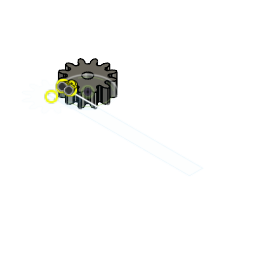
mechtasknipun (Autodesk Fusion 360 design; units mm, degrees)
part number: 2026-02-09-14-14-05-386
description: Spur Gear; Module: 2.1428; Num Teeth: 12; Pressure Angle: 20.0; Backlash: 0.00 mm
part number: 2026-02-09-14-34-28-587
Autodesk Fusion 360 part; units mm, degrees
(part 1 of 2)
sketch "Sketch1" plane through (0, 0, 0) normal (0, 0, 1) x (1, 0, 0)
  circle A0 centre (0, 0) radius 15
  dimension "d1" = 30
  constraint coincident A0.centre origin
  measures "d1" diameter of A0
sketch "Sketch1 (2)" plane through (0, 0, 0) normal (0, 0, 1) x (1, 0, 0) in component "Spur Gear (12 teeth)"
  circle A0 centre (0, 0) radius 10.2346
  circle A1 centre (0, 0) radius 3
extrude "Extrude1" add sketch "Sketch1 (2)" along normal blind 10 makes body 1 in component "Spur Gear (12 teeth)"
sketch "Sketch2" plane through (0, 0, 0) normal (0, 0, 1) x (1, 0, 0) in component "Spur Gear (12 teeth)"
  spline S0 degree 5 poles (11.9532, -1.7553) (11.9618, -1.7565) (11.979, -1.7588) (12.0048, -1.7613) (12.0394, -1.7631) (12.0828, -1.7633) (12.1263, -1.7619) (12.1699, -1.7595) (12.2135, -1.7567) (12.2572, -1.7535) (12.301, -1.7499) (12.3447, -1.7458) (12.3885, -1.741) (12.4324, -1.7355) (12.4763, -1.7292) (12.5202, -1.7222) (12.5641, -1.7147) (12.6081, -1.7066) (12.652, -1.698) (12.696, -1.6891) (12.74, -1.6797) (12.7839, -1.6698) (12.8279, -1.6595) (12.8719, -1.6487) (12.9159, -1.6374) (12.9598, -1.6257) (13.0038, -1.6135) (13.0477, -1.6009) (13.0916, -1.5879) (13.1355, -1.5745) (13.1794, -1.5607) (13.2233, -1.5466) (13.2671, -1.532) (13.311, -1.517) (13.3548, -1.5016) (13.3985, -1.4859) (13.4423, -1.4697) (13.486, -1.4532) (13.5297, -1.4364) (13.5733, -1.4192) (13.6169, -1.4016) (13.6605, -1.3836) (13.704, -1.3654) (13.7475, -1.3467) (13.791, -1.3277) (13.8344, -1.3084) (13.8778, -1.2887) (13.9211, -1.2687) (13.9643, -1.2483) (14.0076, -1.2277) (14.0507, -1.2066) (14.0939, -1.1853) (14.1369, -1.1636) (14.1799, -1.1416) (14.2229, -1.1193) (14.2658, -1.0967) (14.3086, -1.0738) (14.3514, -1.0505) (14.3941, -1.0269) (14.4367, -1.003) (14.4793, -0.9788) (14.5218, -0.9543) (14.5643, -0.9295) (14.6067, -0.9044) (14.649, -0.879) (14.6912, -0.8533) (14.7334, -0.8273) (14.7755, -0.801) (14.8175, -0.7744) (14.8595, -0.7475) (14.9014, -0.7203) (14.9348, -0.6983) (14.9598, -0.6817) (14.9765, -0.6706) (14.9849, -0.665) knots 0 0 0 0 0 0 0.01428571 0.02857143 0.04285714 0.05714286 0.07142857 0.08571429 0.1 0.11428571 0.12857143 0.14285714 0.15714286 0.17142857 0.18571429 0.2 0.21428571 0.22857143 0.24285714 0.25714286 0.27142857 0.28571429 0.3 0.31428571 0.32857143 0.34285714 0.35714286 0.37142857 0.38571429 0.4 0.41428571 0.42857143 0.44285714 0.45714286 0.47142857 0.48571429 0.5 0.51428571 0.52857143 0.54285714 0.55714286 0.57142857 0.58571429 0.6 0.61428571 0.62857143 0.64285714 0.65714286 0.67142857 0.68571429 0.7 0.71428571 0.72857143 0.74285714 0.75714286 0.77142857 0.78571429 0.8 0.81428571 0.82857143 0.84285714 0.85714286 0.87142857 0.88571429 0.9 0.91428571 0.92857143 0.94285714 0.95714286 0.97142857 0.98571429 1 1 1 1 1 1
  spline S1 degree 5 poles (11.9532, 1.7553) (11.9618, 1.7565) (11.979, 1.7588) (12.0048, 1.7613) (12.0394, 1.7631) (12.0828, 1.7633) (12.1263, 1.7619) (12.1699, 1.7595) (12.2135, 1.7567) (12.2572, 1.7535) (12.301, 1.7499) (12.3447, 1.7458) (12.3885, 1.741) (12.4324, 1.7355) (12.4763, 1.7292) (12.5202, 1.7222) (12.5641, 1.7147) (12.6081, 1.7066) (12.652, 1.698) (12.696, 1.6891) (12.74, 1.6797) (12.7839, 1.6698) (12.8279, 1.6595) (12.8719, 1.6487) (12.9159, 1.6374) (12.9598, 1.6257) (13.0038, 1.6135) (13.0477, 1.6009) (13.0916, 1.5879) (13.1355, 1.5745) (13.1794, 1.5607) (13.2233, 1.5466) (13.2671, 1.532) (13.311, 1.517) (13.3548, 1.5016) (13.3985, 1.4859) (13.4423, 1.4697) (13.486, 1.4532) (13.5297, 1.4364) (13.5733, 1.4192) (13.6169, 1.4016) (13.6605, 1.3836) (13.704, 1.3654) (13.7475, 1.3467) (13.791, 1.3277) (13.8344, 1.3084) (13.8778, 1.2887) (13.9211, 1.2687) (13.9643, 1.2483) (14.0076, 1.2277) (14.0507, 1.2066) (14.0939, 1.1853) (14.1369, 1.1636) (14.1799, 1.1416) (14.2229, 1.1193) (14.2658, 1.0967) (14.3086, 1.0738) (14.3514, 1.0505) (14.3941, 1.0269) (14.4367, 1.003) (14.4793, 0.9788) (14.5218, 0.9543) (14.5643, 0.9295) (14.6067, 0.9044) (14.649, 0.879) (14.6912, 0.8533) (14.7334, 0.8273) (14.7755, 0.801) (14.8175, 0.7744) (14.8595, 0.7475) (14.9014, 0.7203) (14.9348, 0.6983) (14.9598, 0.6817) (14.9765, 0.6706) (14.9849, 0.665) knots 0 0 0 0 0 0 0.01428571 0.02857143 0.04285714 0.05714286 0.07142857 0.08571429 0.1 0.11428571 0.12857143 0.14285714 0.15714286 0.17142857 0.18571429 0.2 0.21428571 0.22857143 0.24285714 0.25714286 0.27142857 0.28571429 0.3 0.31428571 0.32857143 0.34285714 0.35714286 0.37142857 0.38571429 0.4 0.41428571 0.42857143 0.44285714 0.45714286 0.47142857 0.48571429 0.5 0.51428571 0.52857143 0.54285714 0.55714286 0.57142857 0.58571429 0.6 0.61428571 0.62857143 0.64285714 0.65714286 0.67142857 0.68571429 0.7 0.71428571 0.72857143 0.74285714 0.75714286 0.77142857 0.78571429 0.8 0.81428571 0.82857143 0.84285714 0.85714286 0.87142857 0.88571429 0.9 0.91428571 0.92857143 0.94285714 0.95714286 0.97142857 0.98571429 1 1 1 1 1 1
  arc A0 (14.9849, -0.665) -> (14.9849, 0.665) centre (0, 0) ccw
  line L0 (10.1162, -1.487) -> (11.9532, -1.7553)
  line L1 (10.1162, 1.487) -> (11.9532, 1.7553)
  line L2 (10.1162, -1.487) -> (10.1162, 1.487)
  point P0 (12.1632, -1.7598)
  point P1 (12.3763, -1.7422)
  point P2 (12.5912, -1.7096)
  point P3 (12.8075, -1.6642)
  point P4 (13.0248, -1.6074)
  point P5 (13.2428, -1.54)
  point P6 (13.4613, -1.4625)
  point P7 (13.68, -1.3754)
  point P8 (13.8987, -1.279)
  point P9 (14.1171, -1.1735)
  point P10 (14.3352, -1.0592)
  point P11 (14.5526, -0.9363)
  point P12 (14.7692, -0.8048)
  point P13 (12.1632, 1.7598)
  point P14 (12.3763, 1.7422)
  point P15 (12.5912, 1.7096)
  point P16 (12.8075, 1.6642)
  point P17 (13.0248, 1.6074)
  point P18 (13.2428, 1.54)
  point P19 (13.4613, 1.4625)
  point P20 (13.68, 1.3754)
  point P21 (13.8987, 1.279)
  point P22 (14.1171, 1.1735)
  point P23 (14.3352, 1.0592)
  point P24 (14.5526, 0.9363)
  point P25 (14.7692, 0.8048)
extrude "Extrude2" add sketch "Sketch2" along normal blind 10 bodies 1 in component "Spur Gear (12 teeth)"
fillet "Fillet1" radius 0.9 2 edges at (10.1258, -1.4884, 5) (10.1258, 1.4884, 5) on bodies 1 in component "Spur Gear (12 teeth)"
pattern_circular "C-Pattern1" count 12 over 360 about axis through (0, 0, 0) along (0, 0, 1) of "Extrude2", "Fillet1" in component "Spur Gear (12 teeth)"
sketch "Sketch3" plane through (0, 0, 0) normal (0, 0, 1) x (1, 0, 0) in component "Spur Gear (12 teeth)"
  circle A0 centre (0, 0) radius 12.8568 construction
copy_body "CopyPasteBodies1" bodies 1 makes body 2
move_body "Move1" bodies 2 to x (1, 0, 0) y (0, 1, 0) z (0, 0, 1) at (0, 0, 0)
sketch "Sketch2 (2)" plane through (0, 0, 10) normal (0, 0, 1) x (-1, 0, 0)
  arc A0 (-9.7871, 28.7076) -> (-9.9726, 28.0156) centre (0, 25.7143) ccw
  arc A1 (-10.9796, 27.3274) -> (-9.9726, 28.0156) centre (-10.8495, 28.2179) ccw
  line L0 (-10.9796, 27.3274) -> (-11.9532, 27.4696)
  spline S0 degree 5 poles (-11.9532, 27.4696) (-11.9618, 27.4708) (-11.979, 27.4731) (-12.0048, 27.4756) (-12.0394, 27.4774) (-12.0828, 27.4775) (-12.1263, 27.4762) (-12.1699, 27.4738) (-12.2135, 27.471) (-12.2572, 27.4677) (-12.301, 27.4642) (-12.3447, 27.4601) (-12.3885, 27.4553) (-12.4324, 27.4498) (-12.4763, 27.4435) (-12.5202, 27.4365) (-12.5641, 27.4289) (-12.6081, 27.4208) (-12.652, 27.4123) (-12.696, 27.4033) (-12.74, 27.394) (-12.7839, 27.3841) (-12.8279, 27.3738) (-12.8719, 27.363) (-12.9159, 27.3517) (-12.9598, 27.34) (-13.0038, 27.3278) (-13.0477, 27.3152) (-13.0916, 27.3022) (-13.1355, 27.2888) (-13.1794, 27.275) (-13.2233, 27.2608) (-13.2671, 27.2463) (-13.311, 27.2313) (-13.3548, 27.2159) (-13.3985, 27.2002) (-13.4423, 27.184) (-13.486, 27.1675) (-13.5297, 27.1507) (-13.5733, 27.1334) (-13.6169, 27.1159) (-13.6605, 27.0979) (-13.704, 27.0796) (-13.7475, 27.061) (-13.791, 27.042) (-13.8344, 27.0227) (-13.8778, 27.003) (-13.9211, 26.983) (-13.9643, 26.9626) (-14.0076, 26.9419) (-14.0507, 26.9209) (-14.0939, 26.8996) (-14.1369, 26.8779) (-14.1799, 26.8559) (-14.2229, 26.8336) (-14.2658, 26.811) (-14.3086, 26.788) (-14.3514, 26.7648) (-14.3941, 26.7412) (-14.4367, 26.7173) (-14.4793, 26.6931) (-14.5218, 26.6686) (-14.5643, 26.6438) (-14.6067, 26.6187) (-14.649, 26.5933) (-14.6912, 26.5676) (-14.7334, 26.5416) (-14.7755, 26.5153) (-14.8175, 26.4887) (-14.8595, 26.4618) (-14.9014, 26.4346) (-14.9348, 26.4126) (-14.9598, 26.396) (-14.9765, 26.3849) (-14.9849, 26.3793) knots 0 0 0 0 0 0 0.01428571 0.02857143 0.04285714 0.05714286 0.07142857 0.08571429 0.1 0.11428571 0.12857143 0.14285714 0.15714286 0.17142857 0.18571429 0.2 0.21428571 0.22857143 0.24285714 0.25714286 0.27142857 0.28571429 0.3 0.31428571 0.32857143 0.34285714 0.35714286 0.37142857 0.38571429 0.4 0.41428571 0.42857143 0.44285714 0.45714286 0.47142857 0.48571429 0.5 0.51428571 0.52857143 0.54285714 0.55714286 0.57142857 0.58571429 0.6 0.61428571 0.62857143 0.64285714 0.65714286 0.67142857 0.68571429 0.7 0.71428571 0.72857143 0.74285714 0.75714286 0.77142857 0.78571429 0.8 0.81428571 0.82857143 0.84285714 0.85714286 0.87142857 0.88571429 0.9 0.91428571 0.92857143 0.94285714 0.95714286 0.97142857 0.98571429 1 1 1 1 1 1
  arc A2 (-14.9849, 26.3793) -> (-14.9849, 25.0493) centre (0, 25.7143) ccw
  spline S1 degree 5 poles (-14.9849, 25.0493) (-14.9765, 25.0437) (-14.9598, 25.0326) (-14.9348, 25.0159) (-14.9014, 24.994) (-14.8595, 24.9668) (-14.8175, 24.9399) (-14.7755, 24.9133) (-14.7334, 24.887) (-14.6912, 24.861) (-14.649, 24.8353) (-14.6067, 24.8099) (-14.5643, 24.7847) (-14.5218, 24.7599) (-14.4793, 24.7354) (-14.4367, 24.7112) (-14.3941, 24.6874) (-14.3514, 24.6638) (-14.3086, 24.6405) (-14.2658, 24.6176) (-14.2229, 24.5949) (-14.1799, 24.5726) (-14.1369, 24.5506) (-14.0939, 24.529) (-14.0507, 24.5076) (-14.0076, 24.4866) (-13.9643, 24.4659) (-13.9211, 24.4456) (-13.8778, 24.4256) (-13.8344, 24.4059) (-13.791, 24.3866) (-13.7475, 24.3676) (-13.704, 24.3489) (-13.6605, 24.3306) (-13.6169, 24.3127) (-13.5733, 24.2951) (-13.5297, 24.2779) (-13.486, 24.261) (-13.4423, 24.2445) (-13.3985, 24.2284) (-13.3548, 24.2127) (-13.311, 24.1973) (-13.2671, 24.1823) (-13.2233, 24.1677) (-13.1794, 24.1535) (-13.1355, 24.1398) (-13.0916, 24.1264) (-13.0477, 24.1134) (-13.0038, 24.1008) (-12.9598, 24.0886) (-12.9159, 24.0768) (-12.8719, 24.0656) (-12.8279, 24.0548) (-12.7839, 24.0445) (-12.74, 24.0346) (-12.696, 24.0252) (-12.652, 24.0163) (-12.6081, 24.0077) (-12.5641, 23.9996) (-12.5202, 23.992) (-12.4763, 23.9851) (-12.4324, 23.9788) (-12.3885, 23.9733) (-12.3447, 23.9685) (-12.301, 23.9644) (-12.2572, 23.9608) (-12.2135, 23.9576) (-12.1699, 23.9548) (-12.1263, 23.9524) (-12.0828, 23.951) (-12.0394, 23.9512) (-12.0048, 23.953) (-11.979, 23.9555) (-11.9618, 23.9577) (-11.9532, 23.959) knots -1 -1 -1 -1 -1 -1 -0.98571429 -0.97142857 -0.95714286 -0.94285714 -0.92857143 -0.91428571 -0.9 -0.88571429 -0.87142857 -0.85714286 -0.84285714 -0.82857143 -0.81428571 -0.8 -0.78571429 -0.77142857 -0.75714286 -0.74285714 -0.72857143 -0.71428571 -0.7 -0.68571429 -0.67142857 -0.65714286 -0.64285714 -0.62857143 -0.61428571 -0.6 -0.58571429 -0.57142857 -0.55714286 -0.54285714 -0.52857143 -0.51428571 -0.5 -0.48571429 -0.47142857 -0.45714286 -0.44285714 -0.42857143 -0.41428571 -0.4 -0.38571429 -0.37142857 -0.35714286 -0.34285714 -0.32857143 -0.31428571 -0.3 -0.28571429 -0.27142857 -0.25714286 -0.24285714 -0.22857143 -0.21428571 -0.2 -0.18571429 -0.17142857 -0.15714286 -0.14285714 -0.12857143 -0.11428571 -0.1 -0.08571429 -0.07142857 -0.05714286 -0.04285714 -0.02857143 -0.01428571 0 0 0 0 0 0
  line L1 (-11.9532, 23.959) -> (-10.9796, 24.1012)
  arc A3 (-9.9726, 23.413) -> (-10.9796, 24.1012) centre (-10.8495, 23.2107) ccw
  arc A4 (-9.9726, 23.413) -> (-9.7871, 22.721) centre (0, 25.7143) ccw
  arc A5 (-10.3151, 21.6215) -> (-9.7871, 22.721) centre (-10.6478, 22.4577) ccw
  line L2 (-10.3151, 21.6215) -> (-11.2295, 21.2578)
  spline S2 degree 5 poles (-11.2295, 21.2578) (-11.2375, 21.2546) (-11.2535, 21.2479) (-11.2771, 21.2372) (-11.308, 21.2215) (-11.3456, 21.1999) (-11.3826, 21.177) (-11.4192, 21.1532) (-11.4556, 21.1289) (-11.4918, 21.1042) (-11.5279, 21.0792) (-11.5637, 21.0538) (-11.5993, 21.0278) (-11.6345, 21.0011) (-11.6694, 20.9737) (-11.7039, 20.9457) (-11.7382, 20.9172) (-11.7722, 20.8882) (-11.806, 20.8588) (-11.8396, 20.8291) (-11.873, 20.7989) (-11.9061, 20.7684) (-11.9391, 20.7375) (-11.9717, 20.7062) (-12.0042, 20.6744) (-12.0364, 20.6423) (-12.0684, 20.6098) (-12.1001, 20.5769) (-12.1316, 20.5437) (-12.163, 20.5101) (-12.1941, 20.4762) (-12.225, 20.442) (-12.2557, 20.4074) (-12.2861, 20.3726) (-12.3164, 20.3373) (-12.3464, 20.3018) (-12.3762, 20.266) (-12.4058, 20.2298) (-12.4352, 20.1934) (-12.4644, 20.1567) (-12.4934, 20.1196) (-12.5222, 20.0823) (-12.5507, 20.0447) (-12.5791, 20.0068) (-12.6072, 19.9686) (-12.6351, 19.9302) (-12.6628, 19.8915) (-12.6904, 19.8525) (-12.7176, 19.8132) (-12.7447, 19.7737) (-12.7716, 19.7339) (-12.7983, 19.6939) (-12.8247, 19.6536) (-12.851, 19.613) (-12.877, 19.5722) (-12.9029, 19.5312) (-12.9285, 19.4899) (-12.9539, 19.4484) (-12.9791, 19.4066) (-13.0041, 19.3646) (-13.0289, 19.3223) (-13.0535, 19.2799) (-13.0778, 19.2371) (-13.102, 19.1942) (-13.1259, 19.151) (-13.1496, 19.1077) (-13.1732, 19.064) (-13.1965, 19.0202) (-13.2196, 18.9762) (-13.2424, 18.9319) (-13.2651, 18.8874) (-13.2831, 18.8517) (-13.2965, 18.8248) (-13.3053, 18.8068) (-13.3098, 18.7978) knots 0 0 0 0 0 0 0.01428571 0.02857143 0.04285714 0.05714286 0.07142857 0.08571429 0.1 0.11428571 0.12857143 0.14285714 0.15714286 0.17142857 0.18571429 0.2 0.21428571 0.22857143 0.24285714 0.25714286 0.27142857 0.28571429 0.3 0.31428571 0.32857143 0.34285714 0.35714286 0.37142857 0.38571429 0.4 0.41428571 0.42857143 0.44285714 0.45714286 0.47142857 0.48571429 0.5 0.51428571 0.52857143 0.54285714 0.55714286 0.57142857 0.58571429 0.6 0.61428571 0.62857143 0.64285714 0.65714286 0.67142857 0.68571429 0.7 0.71428571 0.72857143 0.74285714 0.75714286 0.77142857 0.78571429 0.8 0.81428571 0.82857143 0.84285714 0.85714286 0.87142857 0.88571429 0.9 0.91428571 0.92857143 0.94285714 0.95714286 0.97142857 0.98571429 1 1 1 1 1 1
  arc A6 (-13.3098, 18.7978) -> (-12.6448, 17.6459) centre (0, 25.7143) ccw
  spline S3 degree 5 poles (-12.6448, 17.6459) (-12.6347, 17.6453) (-12.6147, 17.644) (-12.5847, 17.6421) (-12.5448, 17.6398) (-12.4949, 17.6372) (-12.4452, 17.6349) (-12.3955, 17.6328) (-12.3459, 17.6311) (-12.2963, 17.6297) (-12.2469, 17.6285) (-12.1975, 17.6277) (-12.1483, 17.6271) (-12.0991, 17.6269) (-12.05, 17.6269) (-12.0011, 17.6273) (-11.9522, 17.6279) (-11.9034, 17.6288) (-11.8547, 17.6301) (-11.8062, 17.6316) (-11.7577, 17.6335) (-11.7093, 17.6356) (-11.6611, 17.6381) (-11.613, 17.6409) (-11.565, 17.6439) (-11.5171, 17.6473) (-11.4693, 17.651) (-11.4217, 17.655) (-11.3741, 17.6594) (-11.3267, 17.664) (-11.2795, 17.669) (-11.2324, 17.6742) (-11.1854, 17.6798) (-11.1385, 17.6858) (-11.0918, 17.692) (-11.0453, 17.6986) (-10.9989, 17.7055) (-10.9526, 17.7127) (-10.9065, 17.7203) (-10.8605, 17.7282) (-10.8148, 17.7365) (-10.7691, 17.745) (-10.7237, 17.754) (-10.6784, 17.7633) (-10.6334, 17.7729) (-10.5884, 17.7829) (-10.5437, 17.7933) (-10.4992, 17.804) (-10.4548, 17.815) (-10.4107, 17.8265) (-10.3667, 17.8383) (-10.323, 17.8505) (-10.2795, 17.8631) (-10.2363, 17.8762) (-10.1933, 17.8897) (-10.1505, 17.9035) (-10.108, 17.9177) (-10.0656, 17.9323) (-10.0235, 17.9473) (-9.9817, 17.9627) (-9.9402, 17.9786) (-9.899, 17.9951) (-9.8583, 18.0123) (-9.818, 18.03) (-9.778, 18.0484) (-9.7383, 18.0671) (-9.6989, 18.0862) (-9.6596, 18.1056) (-9.6207, 18.1253) (-9.5823, 18.1459) (-9.5448, 18.1677) (-9.5158, 18.1865) (-9.4947, 18.2016) (-9.481, 18.2122) (-9.4742, 18.2175) knots -1 -1 -1 -1 -1 -1 -0.98571429 -0.97142857 -0.95714286 -0.94285714 -0.92857143 -0.91428571 -0.9 -0.88571429 -0.87142857 -0.85714286 -0.84285714 -0.82857143 -0.81428571 -0.8 -0.78571429 -0.77142857 -0.75714286 -0.74285714 -0.72857143 -0.71428571 -0.7 -0.68571429 -0.67142857 -0.65714286 -0.64285714 -0.62857143 -0.61428571 -0.6 -0.58571429 -0.57142857 -0.55714286 -0.54285714 -0.52857143 -0.51428571 -0.5 -0.48571429 -0.47142857 -0.45714286 -0.44285714 -0.42857143 -0.41428571 -0.4 -0.38571429 -0.37142857 -0.35714286 -0.34285714 -0.32857143 -0.31428571 -0.3 -0.28571429 -0.27142857 -0.25714286 -0.24285714 -0.22857143 -0.21428571 -0.2 -0.18571429 -0.17142857 -0.15714286 -0.14285714 -0.12857143 -0.11428571 -0.1 -0.08571429 -0.07142857 -0.05714286 -0.04285714 -0.02857143 -0.01428571 0 0 0 0 0 0
  line L3 (-9.4742, 18.2175) -> (-8.7021, 18.8275)
  arc A7 (-7.4859, 18.735) -> (-8.7021, 18.8275) centre (-8.1441, 18.1213) ccw
  arc A8 (-7.4859, 18.735) -> (-6.9792, 18.2284) centre (0, 25.7143) ccw
  arc A9 (-6.8868, 17.0122) -> (-6.9792, 18.2284) centre (-7.593, 17.5701) ccw
  line L4 (-6.8868, 17.0122) -> (-7.4967, 16.2401)
  spline S4 degree 5 poles (-7.4967, 16.2401) (-7.5021, 16.2333) (-7.5126, 16.2196) (-7.5277, 16.1985) (-7.5466, 16.1694) (-7.5684, 16.1319) (-7.589, 16.0936) (-7.6087, 16.0546) (-7.6281, 16.0154) (-7.6472, 15.976) (-7.6659, 15.9363) (-7.6842, 15.8963) (-7.702, 15.856) (-7.7192, 15.8153) (-7.7357, 15.7741) (-7.7516, 15.7326) (-7.767, 15.6908) (-7.782, 15.6486) (-7.7966, 15.6063) (-7.8108, 15.5638) (-7.8246, 15.521) (-7.8381, 15.478) (-7.8511, 15.4347) (-7.8638, 15.3913) (-7.876, 15.3475) (-7.8878, 15.3036) (-7.8992, 15.2595) (-7.9103, 15.2151) (-7.921, 15.1706) (-7.9314, 15.1258) (-7.9414, 15.0809) (-7.951, 15.0358) (-7.9603, 14.9906) (-7.9692, 14.9451) (-7.9778, 14.8995) (-7.9861, 14.8537) (-7.994, 14.8078) (-8.0016, 14.7617) (-8.0088, 14.7154) (-8.0157, 14.669) (-8.0223, 14.6225) (-8.0285, 14.5758) (-8.0345, 14.5289) (-8.0401, 14.4819) (-8.0453, 14.4348) (-8.0503, 14.3875) (-8.0549, 14.3401) (-8.0593, 14.2926) (-8.0633, 14.245) (-8.067, 14.1972) (-8.0704, 14.1493) (-8.0734, 14.1013) (-8.0762, 14.0532) (-8.0787, 14.0049) (-8.0808, 13.9566) (-8.0827, 13.9081) (-8.0842, 13.8596) (-8.0854, 13.8109) (-8.0864, 13.7621) (-8.087, 13.7132) (-8.0874, 13.6643) (-8.0874, 13.6152) (-8.0871, 13.566) (-8.0866, 13.5167) (-8.0857, 13.4674) (-8.0846, 13.418) (-8.0832, 13.3684) (-8.0814, 13.3188) (-8.0794, 13.2691) (-8.0771, 13.2194) (-8.0745, 13.1695) (-8.0722, 13.1296) (-8.0703, 13.0996) (-8.069, 13.0795) (-8.0683, 13.0695) knots 0 0 0 0 0 0 0.01428571 0.02857143 0.04285714 0.05714286 0.07142857 0.08571429 0.1 0.11428571 0.12857143 0.14285714 0.15714286 0.17142857 0.18571429 0.2 0.21428571 0.22857143 0.24285714 0.25714286 0.27142857 0.28571429 0.3 0.31428571 0.32857143 0.34285714 0.35714286 0.37142857 0.38571429 0.4 0.41428571 0.42857143 0.44285714 0.45714286 0.47142857 0.48571429 0.5 0.51428571 0.52857143 0.54285714 0.55714286 0.57142857 0.58571429 0.6 0.61428571 0.62857143 0.64285714 0.65714286 0.67142857 0.68571429 0.7 0.71428571 0.72857143 0.74285714 0.75714286 0.77142857 0.78571429 0.8 0.81428571 0.82857143 0.84285714 0.85714286 0.87142857 0.88571429 0.9 0.91428571 0.92857143 0.94285714 0.95714286 0.97142857 0.98571429 1 1 1 1 1 1
  arc A10 (-8.0683, 13.0695) -> (-6.9165, 12.4045) centre (0, 25.7143) ccw
  spline S5 degree 5 poles (-6.9165, 12.4045) (-6.9075, 12.4089) (-6.8895, 12.4178) (-6.8626, 12.4312) (-6.8269, 12.4492) (-6.7824, 12.4718) (-6.7381, 12.4947) (-6.6941, 12.5178) (-6.6502, 12.5411) (-6.6066, 12.5646) (-6.5632, 12.5884) (-6.5201, 12.6123) (-6.4771, 12.6365) (-6.4344, 12.6608) (-6.392, 12.6854) (-6.3497, 12.7102) (-6.3077, 12.7352) (-6.2659, 12.7604) (-6.2244, 12.7858) (-6.1831, 12.8114) (-6.1421, 12.8372) (-6.1013, 12.8633) (-6.0607, 12.8895) (-6.0204, 12.916) (-5.9804, 12.9427) (-5.9406, 12.9695) (-5.9011, 12.9966) (-5.8618, 13.0239) (-5.8228, 13.0514) (-5.7841, 13.0792) (-5.7457, 13.1071) (-5.7075, 13.1352) (-5.6696, 13.1636) (-5.632, 13.1921) (-5.5947, 13.2209) (-5.5576, 13.2499) (-5.5209, 13.279) (-5.4845, 13.3084) (-5.4483, 13.338) (-5.4125, 13.3679) (-5.3769, 13.3979) (-5.3417, 13.4281) (-5.3068, 13.4586) (-5.2723, 13.4893) (-5.2381, 13.5202) (-5.2042, 13.5513) (-5.1706, 13.5826) (-5.1374, 13.6142) (-5.1045, 13.6459) (-5.072, 13.6779) (-5.0399, 13.7101) (-5.0081, 13.7425) (-4.9768, 13.7752) (-4.9459, 13.8081) (-4.9153, 13.8413) (-4.8852, 13.8747) (-4.8555, 13.9083) (-4.8261, 13.9421) (-4.7971, 13.9761) (-4.7686, 14.0104) (-4.7406, 14.0449) (-4.7132, 14.0798) (-4.6865, 14.115) (-4.6605, 14.1506) (-4.635, 14.1864) (-4.6101, 14.2225) (-4.5854, 14.2587) (-4.5611, 14.2951) (-4.5373, 14.3317) (-4.5143, 14.3687) (-4.4928, 14.4063) (-4.4771, 14.4372) (-4.4664, 14.4608) (-4.4597, 14.4768) (-4.4565, 14.4848) knots -1 -1 -1 -1 -1 -1 -0.98571429 -0.97142857 -0.95714286 -0.94285714 -0.92857143 -0.91428571 -0.9 -0.88571429 -0.87142857 -0.85714286 -0.84285714 -0.82857143 -0.81428571 -0.8 -0.78571429 -0.77142857 -0.75714286 -0.74285714 -0.72857143 -0.71428571 -0.7 -0.68571429 -0.67142857 -0.65714286 -0.64285714 -0.62857143 -0.61428571 -0.6 -0.58571429 -0.57142857 -0.55714286 -0.54285714 -0.52857143 -0.51428571 -0.5 -0.48571429 -0.47142857 -0.45714286 -0.44285714 -0.42857143 -0.41428571 -0.4 -0.38571429 -0.37142857 -0.35714286 -0.34285714 -0.32857143 -0.31428571 -0.3 -0.28571429 -0.27142857 -0.25714286 -0.24285714 -0.22857143 -0.21428571 -0.2 -0.18571429 -0.17142857 -0.15714286 -0.14285714 -0.12857143 -0.11428571 -0.1 -0.08571429 -0.07142857 -0.05714286 -0.04285714 -0.02857143 -0.01428571 0 0 0 0 0 0
  line L5 (-4.4565, 14.4848) -> (-4.0928, 15.3991)
  arc A11 (-2.9933, 15.9272) -> (-4.0928, 15.3991) centre (-3.2566, 15.0665) ccw
  arc A12 (-2.9933, 15.9272) -> (-2.3013, 15.7417) centre (0, 25.7143) ccw
  arc A13 (-1.6131, 14.7347) -> (-2.3013, 15.7417) centre (-2.5036, 14.8648) ccw
  line L6 (-1.6131, 14.7347) -> (-1.7553, 13.761)
  spline S6 degree 5 poles (-1.7553, 13.761) (-1.7565, 13.7525) (-1.7588, 13.7353) (-1.7613, 13.7095) (-1.7631, 13.6749) (-1.7633, 13.6315) (-1.7619, 13.588) (-1.7595, 13.5444) (-1.7567, 13.5008) (-1.7535, 13.4571) (-1.7499, 13.4133) (-1.7458, 13.3696) (-1.741, 13.3257) (-1.7355, 13.2819) (-1.7292, 13.238) (-1.7222, 13.1941) (-1.7147, 13.1502) (-1.7066, 13.1062) (-1.698, 13.0622) (-1.6891, 13.0183) (-1.6797, 12.9743) (-1.6698, 12.9303) (-1.6595, 12.8864) (-1.6487, 12.8424) (-1.6374, 12.7984) (-1.6257, 12.7545) (-1.6135, 12.7105) (-1.6009, 12.6666) (-1.5879, 12.6227) (-1.5745, 12.5787) (-1.5607, 12.5349) (-1.5466, 12.491) (-1.532, 12.4471) (-1.517, 12.4033) (-1.5016, 12.3595) (-1.4859, 12.3157) (-1.4697, 12.272) (-1.4532, 12.2283) (-1.4364, 12.1846) (-1.4192, 12.141) (-1.4016, 12.0973) (-1.3836, 12.0538) (-1.3654, 12.0102) (-1.3467, 11.9667) (-1.3277, 11.9233) (-1.3084, 11.8799) (-1.2887, 11.8365) (-1.2687, 11.7932) (-1.2483, 11.7499) (-1.2277, 11.7067) (-1.2066, 11.6636) (-1.1853, 11.6204) (-1.1636, 11.5774) (-1.1416, 11.5344) (-1.1193, 11.4914) (-1.0967, 11.4485) (-1.0738, 11.4057) (-1.0505, 11.3629) (-1.0269, 11.3202) (-1.003, 11.2776) (-0.9788, 11.235) (-0.9543, 11.1924) (-0.9295, 11.15) (-0.9044, 11.1076) (-0.879, 11.0653) (-0.8533, 11.023) (-0.8273, 10.9809) (-0.801, 10.9388) (-0.7744, 10.8968) (-0.7475, 10.8548) (-0.7203, 10.8129) (-0.6983, 10.7795) (-0.6817, 10.7545) (-0.6706, 10.7378) (-0.665, 10.7294) knots 0 0 0 0 0 0 0.01428571 0.02857143 0.04285714 0.05714286 0.07142857 0.08571429 0.1 0.11428571 0.12857143 0.14285714 0.15714286 0.17142857 0.18571429 0.2 0.21428571 0.22857143 0.24285714 0.25714286 0.27142857 0.28571429 0.3 0.31428571 0.32857143 0.34285714 0.35714286 0.37142857 0.38571429 0.4 0.41428571 0.42857143 0.44285714 0.45714286 0.47142857 0.48571429 0.5 0.51428571 0.52857143 0.54285714 0.55714286 0.57142857 0.58571429 0.6 0.61428571 0.62857143 0.64285714 0.65714286 0.67142857 0.68571429 0.7 0.71428571 0.72857143 0.74285714 0.75714286 0.77142857 0.78571429 0.8 0.81428571 0.82857143 0.84285714 0.85714286 0.87142857 0.88571429 0.9 0.91428571 0.92857143 0.94285714 0.95714286 0.97142857 0.98571429 1 1 1 1 1 1
  arc A14 (-0.665, 10.7294) -> (0.665, 10.7294) centre (0, 25.7143) ccw
  spline S7 degree 5 poles (0.665, 10.7294) (0.6706, 10.7378) (0.6817, 10.7545) (0.6983, 10.7795) (0.7203, 10.8129) (0.7475, 10.8548) (0.7744, 10.8968) (0.801, 10.9388) (0.8273, 10.9809) (0.8533, 11.023) (0.879, 11.0653) (0.9044, 11.1076) (0.9295, 11.15) (0.9543, 11.1924) (0.9788, 11.235) (1.003, 11.2776) (1.0269, 11.3202) (1.0505, 11.3629) (1.0738, 11.4057) (1.0967, 11.4485) (1.1193, 11.4914) (1.1416, 11.5344) (1.1636, 11.5774) (1.1853, 11.6204) (1.2066, 11.6636) (1.2277, 11.7067) (1.2483, 11.7499) (1.2687, 11.7932) (1.2887, 11.8365) (1.3084, 11.8799) (1.3277, 11.9233) (1.3467, 11.9667) (1.3654, 12.0102) (1.3836, 12.0538) (1.4016, 12.0973) (1.4192, 12.141) (1.4364, 12.1846) (1.4532, 12.2283) (1.4697, 12.272) (1.4859, 12.3157) (1.5016, 12.3595) (1.517, 12.4033) (1.532, 12.4471) (1.5466, 12.491) (1.5607, 12.5349) (1.5745, 12.5787) (1.5879, 12.6227) (1.6009, 12.6666) (1.6135, 12.7105) (1.6257, 12.7545) (1.6374, 12.7984) (1.6487, 12.8424) (1.6595, 12.8864) (1.6698, 12.9303) (1.6797, 12.9743) (1.6891, 13.0183) (1.698, 13.0622) (1.7066, 13.1062) (1.7147, 13.1502) (1.7222, 13.1941) (1.7292, 13.238) (1.7355, 13.2819) (1.741, 13.3257) (1.7458, 13.3696) (1.7499, 13.4133) (1.7535, 13.4571) (1.7567, 13.5008) (1.7595, 13.5444) (1.7619, 13.588) (1.7633, 13.6315) (1.7631, 13.6749) (1.7613, 13.7095) (1.7588, 13.7353) (1.7565, 13.7525) (1.7553, 13.761) knots -1 -1 -1 -1 -1 -1 -0.98571429 -0.97142857 -0.95714286 -0.94285714 -0.92857143 -0.91428571 -0.9 -0.88571429 -0.87142857 -0.85714286 -0.84285714 -0.82857143 -0.81428571 -0.8 -0.78571429 -0.77142857 -0.75714286 -0.74285714 -0.72857143 -0.71428571 -0.7 -0.68571429 -0.67142857 -0.65714286 -0.64285714 -0.62857143 -0.61428571 -0.6 -0.58571429 -0.57142857 -0.55714286 -0.54285714 -0.52857143 -0.51428571 -0.5 -0.48571429 -0.47142857 -0.45714286 -0.44285714 -0.42857143 -0.41428571 -0.4 -0.38571429 -0.37142857 -0.35714286 -0.34285714 -0.32857143 -0.31428571 -0.3 -0.28571429 -0.27142857 -0.25714286 -0.24285714 -0.22857143 -0.21428571 -0.2 -0.18571429 -0.17142857 -0.15714286 -0.14285714 -0.12857143 -0.11428571 -0.1 -0.08571429 -0.07142857 -0.05714286 -0.04285714 -0.02857143 -0.01428571 0 0 0 0 0 0
  line L7 (1.7553, 13.761) -> (1.6131, 14.7347)
  arc A15 (2.3013, 15.7417) -> (1.6131, 14.7347) centre (2.5036, 14.8648) ccw
  arc A16 (2.3013, 15.7417) -> (2.9933, 15.9272) centre (0, 25.7143) ccw
  arc A17 (4.0928, 15.3991) -> (2.9933, 15.9272) centre (3.2566, 15.0665) ccw
  line L8 (4.0928, 15.3991) -> (4.4565, 14.4848)
  spline S8 degree 5 poles (4.4565, 14.4848) (4.4597, 14.4768) (4.4664, 14.4608) (4.4771, 14.4372) (4.4928, 14.4063) (4.5143, 14.3687) (4.5373, 14.3317) (4.5611, 14.2951) (4.5854, 14.2587) (4.6101, 14.2225) (4.635, 14.1864) (4.6605, 14.1506) (4.6865, 14.115) (4.7132, 14.0798) (4.7406, 14.0449) (4.7686, 14.0104) (4.7971, 13.9761) (4.8261, 13.9421) (4.8555, 13.9083) (4.8852, 13.8747) (4.9153, 13.8413) (4.9459, 13.8081) (4.9768, 13.7752) (5.0081, 13.7425) (5.0399, 13.7101) (5.072, 13.6779) (5.1045, 13.6459) (5.1374, 13.6142) (5.1706, 13.5826) (5.2042, 13.5513) (5.2381, 13.5202) (5.2723, 13.4893) (5.3068, 13.4586) (5.3417, 13.4281) (5.3769, 13.3979) (5.4125, 13.3679) (5.4483, 13.338) (5.4845, 13.3084) (5.5209, 13.279) (5.5576, 13.2499) (5.5947, 13.2209) (5.632, 13.1921) (5.6696, 13.1636) (5.7075, 13.1352) (5.7457, 13.1071) (5.7841, 13.0792) (5.8228, 13.0514) (5.8618, 13.0239) (5.9011, 12.9966) (5.9406, 12.9695) (5.9804, 12.9427) (6.0204, 12.916) (6.0607, 12.8895) (6.1013, 12.8633) (6.1421, 12.8372) (6.1831, 12.8114) (6.2244, 12.7858) (6.2659, 12.7604) (6.3077, 12.7352) (6.3497, 12.7102) (6.392, 12.6854) (6.4344, 12.6608) (6.4771, 12.6365) (6.5201, 12.6123) (6.5632, 12.5884) (6.6066, 12.5646) (6.6502, 12.5411) (6.6941, 12.5178) (6.7381, 12.4947) (6.7824, 12.4718) (6.8269, 12.4492) (6.8626, 12.4312) (6.8895, 12.4178) (6.9075, 12.4089) (6.9165, 12.4045) knots 0 0 0 0 0 0 0.01428571 0.02857143 0.04285714 0.05714286 0.07142857 0.08571429 0.1 0.11428571 0.12857143 0.14285714 0.15714286 0.17142857 0.18571429 0.2 0.21428571 0.22857143 0.24285714 0.25714286 0.27142857 0.28571429 0.3 0.31428571 0.32857143 0.34285714 0.35714286 0.37142857 0.38571429 0.4 0.41428571 0.42857143 0.44285714 0.45714286 0.47142857 0.48571429 0.5 0.51428571 0.52857143 0.54285714 0.55714286 0.57142857 0.58571429 0.6 0.61428571 0.62857143 0.64285714 0.65714286 0.67142857 0.68571429 0.7 0.71428571 0.72857143 0.74285714 0.75714286 0.77142857 0.78571429 0.8 0.81428571 0.82857143 0.84285714 0.85714286 0.87142857 0.88571429 0.9 0.91428571 0.92857143 0.94285714 0.95714286 0.97142857 0.98571429 1 1 1 1 1 1
  arc A18 (6.9165, 12.4045) -> (8.0683, 13.0695) centre (0, 25.7143) ccw
  spline S9 degree 5 poles (8.0683, 13.0695) (8.069, 13.0795) (8.0703, 13.0996) (8.0722, 13.1296) (8.0745, 13.1695) (8.0771, 13.2194) (8.0794, 13.2691) (8.0814, 13.3188) (8.0832, 13.3684) (8.0846, 13.418) (8.0857, 13.4674) (8.0866, 13.5167) (8.0871, 13.566) (8.0874, 13.6152) (8.0874, 13.6643) (8.087, 13.7132) (8.0864, 13.7621) (8.0854, 13.8109) (8.0842, 13.8596) (8.0827, 13.9081) (8.0808, 13.9566) (8.0787, 14.0049) (8.0762, 14.0532) (8.0734, 14.1013) (8.0704, 14.1493) (8.067, 14.1972) (8.0633, 14.245) (8.0593, 14.2926) (8.0549, 14.3401) (8.0503, 14.3875) (8.0453, 14.4348) (8.0401, 14.4819) (8.0345, 14.5289) (8.0285, 14.5758) (8.0223, 14.6225) (8.0157, 14.669) (8.0088, 14.7154) (8.0016, 14.7617) (7.994, 14.8078) (7.9861, 14.8537) (7.9778, 14.8995) (7.9692, 14.9451) (7.9603, 14.9906) (7.951, 15.0358) (7.9414, 15.0809) (7.9314, 15.1258) (7.921, 15.1706) (7.9103, 15.2151) (7.8992, 15.2595) (7.8878, 15.3036) (7.876, 15.3475) (7.8638, 15.3913) (7.8511, 15.4347) (7.8381, 15.478) (7.8246, 15.521) (7.8108, 15.5638) (7.7966, 15.6063) (7.782, 15.6486) (7.767, 15.6908) (7.7516, 15.7326) (7.7357, 15.7741) (7.7192, 15.8153) (7.702, 15.856) (7.6842, 15.8963) (7.6659, 15.9363) (7.6472, 15.976) (7.6281, 16.0154) (7.6087, 16.0546) (7.589, 16.0936) (7.5684, 16.1319) (7.5466, 16.1694) (7.5277, 16.1985) (7.5126, 16.2196) (7.5021, 16.2333) (7.4967, 16.2401) knots -1 -1 -1 -1 -1 -1 -0.98571429 -0.97142857 -0.95714286 -0.94285714 -0.92857143 -0.91428571 -0.9 -0.88571429 -0.87142857 -0.85714286 -0.84285714 -0.82857143 -0.81428571 -0.8 -0.78571429 -0.77142857 -0.75714286 -0.74285714 -0.72857143 -0.71428571 -0.7 -0.68571429 -0.67142857 -0.65714286 -0.64285714 -0.62857143 -0.61428571 -0.6 -0.58571429 -0.57142857 -0.55714286 -0.54285714 -0.52857143 -0.51428571 -0.5 -0.48571429 -0.47142857 -0.45714286 -0.44285714 -0.42857143 -0.41428571 -0.4 -0.38571429 -0.37142857 -0.35714286 -0.34285714 -0.32857143 -0.31428571 -0.3 -0.28571429 -0.27142857 -0.25714286 -0.24285714 -0.22857143 -0.21428571 -0.2 -0.18571429 -0.17142857 -0.15714286 -0.14285714 -0.12857143 -0.11428571 -0.1 -0.08571429 -0.07142857 -0.05714286 -0.04285714 -0.02857143 -0.01428571 0 0 0 0 0 0
  line L9 (7.4967, 16.2401) -> (6.8868, 17.0122)
  arc A19 (6.9792, 18.2284) -> (6.8868, 17.0122) centre (7.593, 17.5701) ccw
  arc A20 (6.9792, 18.2284) -> (7.4859, 18.735) centre (0, 25.7143) ccw
  arc A21 (8.7021, 18.8275) -> (7.4859, 18.735) centre (8.1441, 18.1213) ccw
  line L10 (8.7021, 18.8275) -> (9.4742, 18.2175)
  spline S10 degree 5 poles (9.4742, 18.2175) (9.481, 18.2122) (9.4947, 18.2016) (9.5158, 18.1865) (9.5448, 18.1677) (9.5823, 18.1459) (9.6207, 18.1253) (9.6596, 18.1056) (9.6989, 18.0862) (9.7383, 18.0671) (9.778, 18.0484) (9.818, 18.03) (9.8583, 18.0123) (9.899, 17.9951) (9.9402, 17.9786) (9.9817, 17.9627) (10.0235, 17.9473) (10.0656, 17.9323) (10.108, 17.9177) (10.1505, 17.9035) (10.1933, 17.8897) (10.2363, 17.8762) (10.2795, 17.8631) (10.323, 17.8505) (10.3667, 17.8383) (10.4107, 17.8265) (10.4548, 17.815) (10.4992, 17.804) (10.5437, 17.7933) (10.5884, 17.7829) (10.6334, 17.7729) (10.6784, 17.7633) (10.7237, 17.754) (10.7691, 17.745) (10.8148, 17.7365) (10.8605, 17.7282) (10.9065, 17.7203) (10.9526, 17.7127) (10.9989, 17.7055) (11.0453, 17.6986) (11.0918, 17.692) (11.1385, 17.6858) (11.1854, 17.6798) (11.2324, 17.6742) (11.2795, 17.669) (11.3267, 17.664) (11.3741, 17.6594) (11.4217, 17.655) (11.4693, 17.651) (11.5171, 17.6473) (11.565, 17.6439) (11.613, 17.6409) (11.6611, 17.6381) (11.7093, 17.6356) (11.7577, 17.6335) (11.8062, 17.6316) (11.8547, 17.6301) (11.9034, 17.6288) (11.9522, 17.6279) (12.0011, 17.6273) (12.05, 17.6269) (12.0991, 17.6269) (12.1483, 17.6271) (12.1975, 17.6277) (12.2469, 17.6285) (12.2963, 17.6297) (12.3459, 17.6311) (12.3955, 17.6328) (12.4452, 17.6349) (12.4949, 17.6372) (12.5448, 17.6398) (12.5847, 17.6421) (12.6147, 17.644) (12.6347, 17.6453) (12.6448, 17.6459) knots 0 0 0 0 0 0 0.01428571 0.02857143 0.04285714 0.05714286 0.07142857 0.08571429 0.1 0.11428571 0.12857143 0.14285714 0.15714286 0.17142857 0.18571429 0.2 0.21428571 0.22857143 0.24285714 0.25714286 0.27142857 0.28571429 0.3 0.31428571 0.32857143 0.34285714 0.35714286 0.37142857 0.38571429 0.4 0.41428571 0.42857143 0.44285714 0.45714286 0.47142857 0.48571429 0.5 0.51428571 0.52857143 0.54285714 0.55714286 0.57142857 0.58571429 0.6 0.61428571 0.62857143 0.64285714 0.65714286 0.67142857 0.68571429 0.7 0.71428571 0.72857143 0.74285714 0.75714286 0.77142857 0.78571429 0.8 0.81428571 0.82857143 0.84285714 0.85714286 0.87142857 0.88571429 0.9 0.91428571 0.92857143 0.94285714 0.95714286 0.97142857 0.98571429 1 1 1 1 1 1
  arc A22 (12.6448, 17.6459) -> (13.3098, 18.7978) centre (0, 25.7143) ccw
  spline S11 degree 5 poles (13.3098, 18.7978) (13.3053, 18.8068) (13.2965, 18.8248) (13.2831, 18.8517) (13.2651, 18.8874) (13.2424, 18.9319) (13.2196, 18.9762) (13.1965, 19.0202) (13.1732, 19.064) (13.1496, 19.1077) (13.1259, 19.151) (13.102, 19.1942) (13.0778, 19.2371) (13.0535, 19.2799) (13.0289, 19.3223) (13.0041, 19.3646) (12.9791, 19.4066) (12.9539, 19.4484) (12.9285, 19.4899) (12.9029, 19.5312) (12.877, 19.5722) (12.851, 19.613) (12.8247, 19.6536) (12.7983, 19.6939) (12.7716, 19.7339) (12.7447, 19.7737) (12.7176, 19.8132) (12.6904, 19.8525) (12.6628, 19.8915) (12.6351, 19.9302) (12.6072, 19.9686) (12.5791, 20.0068) (12.5507, 20.0447) (12.5222, 20.0823) (12.4934, 20.1196) (12.4644, 20.1567) (12.4352, 20.1934) (12.4058, 20.2298) (12.3762, 20.266) (12.3464, 20.3018) (12.3164, 20.3373) (12.2861, 20.3726) (12.2557, 20.4074) (12.225, 20.442) (12.1941, 20.4762) (12.163, 20.5101) (12.1316, 20.5437) (12.1001, 20.5769) (12.0684, 20.6098) (12.0364, 20.6423) (12.0042, 20.6744) (11.9717, 20.7062) (11.9391, 20.7375) (11.9061, 20.7684) (11.873, 20.7989) (11.8396, 20.8291) (11.806, 20.8588) (11.7722, 20.8882) (11.7382, 20.9172) (11.7039, 20.9457) (11.6694, 20.9737) (11.6345, 21.0011) (11.5993, 21.0278) (11.5637, 21.0538) (11.5279, 21.0792) (11.4918, 21.1042) (11.4556, 21.1289) (11.4192, 21.1532) (11.3826, 21.177) (11.3456, 21.1999) (11.308, 21.2215) (11.2771, 21.2372) (11.2535, 21.2479) (11.2375, 21.2546) (11.2295, 21.2578) knots -1 -1 -1 -1 -1 -1 -0.98571429 -0.97142857 -0.95714286 -0.94285714 -0.92857143 -0.91428571 -0.9 -0.88571429 -0.87142857 -0.85714286 -0.84285714 -0.82857143 -0.81428571 -0.8 -0.78571429 -0.77142857 -0.75714286 -0.74285714 -0.72857143 -0.71428571 -0.7 -0.68571429 -0.67142857 -0.65714286 -0.64285714 -0.62857143 -0.61428571 -0.6 -0.58571429 -0.57142857 -0.55714286 -0.54285714 -0.52857143 -0.51428571 -0.5 -0.48571429 -0.47142857 -0.45714286 -0.44285714 -0.42857143 -0.41428571 -0.4 -0.38571429 -0.37142857 -0.35714286 -0.34285714 -0.32857143 -0.31428571 -0.3 -0.28571429 -0.27142857 -0.25714286 -0.24285714 -0.22857143 -0.21428571 -0.2 -0.18571429 -0.17142857 -0.15714286 -0.14285714 -0.12857143 -0.11428571 -0.1 -0.08571429 -0.07142857 -0.05714286 -0.04285714 -0.02857143 -0.01428571 0 0 0 0 0 0
  line L11 (11.2295, 21.2578) -> (10.3151, 21.6215)
  arc A23 (9.7871, 22.721) -> (10.3151, 21.6215) centre (10.6478, 22.4577) ccw
  arc A24 (9.7871, 22.721) -> (9.9726, 23.413) centre (0, 25.7143) ccw
  arc A25 (10.9796, 24.1012) -> (9.9726, 23.413) centre (10.8495, 23.2107) ccw
  line L12 (10.9796, 24.1012) -> (11.9532, 23.959)
  spline S12 degree 5 poles (11.9532, 23.959) (11.9618, 23.9577) (11.979, 23.9555) (12.0048, 23.953) (12.0394, 23.9512) (12.0828, 23.951) (12.1263, 23.9524) (12.1699, 23.9548) (12.2135, 23.9576) (12.2572, 23.9608) (12.301, 23.9644) (12.3447, 23.9685) (12.3885, 23.9733) (12.4324, 23.9788) (12.4763, 23.9851) (12.5202, 23.992) (12.5641, 23.9996) (12.6081, 24.0077) (12.652, 24.0163) (12.696, 24.0252) (12.74, 24.0346) (12.7839, 24.0445) (12.8279, 24.0548) (12.8719, 24.0656) (12.9159, 24.0768) (12.9598, 24.0886) (13.0038, 24.1008) (13.0477, 24.1134) (13.0916, 24.1264) (13.1355, 24.1398) (13.1794, 24.1535) (13.2233, 24.1677) (13.2671, 24.1823) (13.311, 24.1973) (13.3548, 24.2127) (13.3985, 24.2284) (13.4423, 24.2445) (13.486, 24.261) (13.5297, 24.2779) (13.5733, 24.2951) (13.6169, 24.3127) (13.6605, 24.3306) (13.704, 24.3489) (13.7475, 24.3676) (13.791, 24.3866) (13.8344, 24.4059) (13.8778, 24.4256) (13.9211, 24.4456) (13.9643, 24.4659) (14.0076, 24.4866) (14.0507, 24.5076) (14.0939, 24.529) (14.1369, 24.5506) (14.1799, 24.5726) (14.2229, 24.5949) (14.2658, 24.6176) (14.3086, 24.6405) (14.3514, 24.6638) (14.3941, 24.6874) (14.4367, 24.7112) (14.4793, 24.7354) (14.5218, 24.7599) (14.5643, 24.7847) (14.6067, 24.8099) (14.649, 24.8353) (14.6912, 24.861) (14.7334, 24.887) (14.7755, 24.9133) (14.8175, 24.9399) (14.8595, 24.9668) (14.9014, 24.994) (14.9348, 25.0159) (14.9598, 25.0326) (14.9765, 25.0437) (14.9849, 25.0493) knots 0 0 0 0 0 0 0.01428571 0.02857143 0.04285714 0.05714286 0.07142857 0.08571429 0.1 0.11428571 0.12857143 0.14285714 0.15714286 0.17142857 0.18571429 0.2 0.21428571 0.22857143 0.24285714 0.25714286 0.27142857 0.28571429 0.3 0.31428571 0.32857143 0.34285714 0.35714286 0.37142857 0.38571429 0.4 0.41428571 0.42857143 0.44285714 0.45714286 0.47142857 0.48571429 0.5 0.51428571 0.52857143 0.54285714 0.55714286 0.57142857 0.58571429 0.6 0.61428571 0.62857143 0.64285714 0.65714286 0.67142857 0.68571429 0.7 0.71428571 0.72857143 0.74285714 0.75714286 0.77142857 0.78571429 0.8 0.81428571 0.82857143 0.84285714 0.85714286 0.87142857 0.88571429 0.9 0.91428571 0.92857143 0.94285714 0.95714286 0.97142857 0.98571429 1 1 1 1 1 1
  arc A26 (14.9849, 25.0493) -> (14.9849, 26.3793) centre (0, 25.7143) ccw
  spline S13 degree 5 poles (14.9849, 26.3793) (14.9765, 26.3849) (14.9598, 26.396) (14.9348, 26.4126) (14.9014, 26.4346) (14.8595, 26.4618) (14.8175, 26.4887) (14.7755, 26.5153) (14.7334, 26.5416) (14.6912, 26.5676) (14.649, 26.5933) (14.6067, 26.6187) (14.5643, 26.6438) (14.5218, 26.6686) (14.4793, 26.6931) (14.4367, 26.7173) (14.3941, 26.7412) (14.3514, 26.7648) (14.3086, 26.788) (14.2658, 26.811) (14.2229, 26.8336) (14.1799, 26.8559) (14.1369, 26.8779) (14.0939, 26.8996) (14.0507, 26.9209) (14.0076, 26.9419) (13.9643, 26.9626) (13.9211, 26.983) (13.8778, 27.003) (13.8344, 27.0227) (13.791, 27.042) (13.7475, 27.061) (13.704, 27.0796) (13.6605, 27.0979) (13.6169, 27.1159) (13.5733, 27.1334) (13.5297, 27.1507) (13.486, 27.1675) (13.4423, 27.184) (13.3985, 27.2002) (13.3548, 27.2159) (13.311, 27.2313) (13.2671, 27.2463) (13.2233, 27.2608) (13.1794, 27.275) (13.1355, 27.2888) (13.0916, 27.3022) (13.0477, 27.3152) (13.0038, 27.3278) (12.9598, 27.34) (12.9159, 27.3517) (12.8719, 27.363) (12.8279, 27.3738) (12.7839, 27.3841) (12.74, 27.394) (12.696, 27.4033) (12.652, 27.4123) (12.6081, 27.4208) (12.5641, 27.4289) (12.5202, 27.4365) (12.4763, 27.4435) (12.4324, 27.4498) (12.3885, 27.4553) (12.3447, 27.4601) (12.301, 27.4642) (12.2572, 27.4677) (12.2135, 27.471) (12.1699, 27.4738) (12.1263, 27.4762) (12.0828, 27.4775) (12.0394, 27.4774) (12.0048, 27.4756) (11.979, 27.4731) (11.9618, 27.4708) (11.9532, 27.4696) knots -1 -1 -1 -1 -1 -1 -0.98571429 -0.97142857 -0.95714286 -0.94285714 -0.92857143 -0.91428571 -0.9 -0.88571429 -0.87142857 -0.85714286 -0.84285714 -0.82857143 -0.81428571 -0.8 -0.78571429 -0.77142857 -0.75714286 -0.74285714 -0.72857143 -0.71428571 -0.7 -0.68571429 -0.67142857 -0.65714286 -0.64285714 -0.62857143 -0.61428571 -0.6 -0.58571429 -0.57142857 -0.55714286 -0.54285714 -0.52857143 -0.51428571 -0.5 -0.48571429 -0.47142857 -0.45714286 -0.44285714 -0.42857143 -0.41428571 -0.4 -0.38571429 -0.37142857 -0.35714286 -0.34285714 -0.32857143 -0.31428571 -0.3 -0.28571429 -0.27142857 -0.25714286 -0.24285714 -0.22857143 -0.21428571 -0.2 -0.18571429 -0.17142857 -0.15714286 -0.14285714 -0.12857143 -0.11428571 -0.1 -0.08571429 -0.07142857 -0.05714286 -0.04285714 -0.02857143 -0.01428571 0 0 0 0 0 0
  line L13 (11.9532, 27.4696) -> (10.9796, 27.3274)
  arc A27 (9.9726, 28.0156) -> (10.9796, 27.3274) centre (10.8495, 28.2179) ccw
  arc A28 (9.9726, 28.0156) -> (9.7871, 28.7076) centre (0, 25.7143) ccw
  arc A29 (10.3151, 29.8071) -> (9.7871, 28.7076) centre (10.6478, 28.9708) ccw
  line L14 (10.3151, 29.8071) -> (11.2295, 30.1708)
  spline S14 degree 5 poles (11.2295, 30.1708) (11.2375, 30.174) (11.2535, 30.1806) (11.2771, 30.1914) (11.308, 30.2071) (11.3456, 30.2286) (11.3826, 30.2516) (11.4192, 30.2754) (11.4556, 30.2997) (11.4918, 30.3244) (11.5279, 30.3493) (11.5637, 30.3748) (11.5993, 30.4008) (11.6345, 30.4275) (11.6694, 30.4549) (11.7039, 30.4829) (11.7382, 30.5114) (11.7722, 30.5404) (11.806, 30.5698) (11.8396, 30.5995) (11.873, 30.6296) (11.9061, 30.6601) (11.9391, 30.6911) (11.9717, 30.7224) (12.0042, 30.7541) (12.0364, 30.7863) (12.0684, 30.8188) (12.1001, 30.8517) (12.1316, 30.8849) (12.163, 30.9185) (12.1941, 30.9524) (12.225, 30.9866) (12.2557, 31.0211) (12.2861, 31.056) (12.3164, 31.0912) (12.3464, 31.1268) (12.3762, 31.1626) (12.4058, 31.1987) (12.4352, 31.2352) (12.4644, 31.2719) (12.4934, 31.309) (12.5222, 31.3463) (12.5507, 31.3839) (12.5791, 31.4218) (12.6072, 31.4599) (12.6351, 31.4984) (12.6628, 31.5371) (12.6904, 31.5761) (12.7176, 31.6154) (12.7447, 31.6549) (12.7716, 31.6947) (12.7983, 31.7347) (12.8247, 31.775) (12.851, 31.8155) (12.877, 31.8563) (12.9029, 31.8974) (12.9285, 31.9387) (12.9539, 31.9802) (12.9791, 32.022) (13.0041, 32.064) (13.0289, 32.1062) (13.0535, 32.1487) (13.0778, 32.1914) (13.102, 32.2344) (13.1259, 32.2775) (13.1496, 32.3209) (13.1732, 32.3645) (13.1965, 32.4084) (13.2196, 32.4524) (13.2424, 32.4967) (13.2651, 32.5411) (13.2831, 32.5769) (13.2965, 32.6038) (13.3053, 32.6218) (13.3098, 32.6308) knots 0 0 0 0 0 0 0.01428571 0.02857143 0.04285714 0.05714286 0.07142857 0.08571429 0.1 0.11428571 0.12857143 0.14285714 0.15714286 0.17142857 0.18571429 0.2 0.21428571 0.22857143 0.24285714 0.25714286 0.27142857 0.28571429 0.3 0.31428571 0.32857143 0.34285714 0.35714286 0.37142857 0.38571429 0.4 0.41428571 0.42857143 0.44285714 0.45714286 0.47142857 0.48571429 0.5 0.51428571 0.52857143 0.54285714 0.55714286 0.57142857 0.58571429 0.6 0.61428571 0.62857143 0.64285714 0.65714286 0.67142857 0.68571429 0.7 0.71428571 0.72857143 0.74285714 0.75714286 0.77142857 0.78571429 0.8 0.81428571 0.82857143 0.84285714 0.85714286 0.87142857 0.88571429 0.9 0.91428571 0.92857143 0.94285714 0.95714286 0.97142857 0.98571429 1 1 1 1 1 1
  arc A30 (13.3098, 32.6308) -> (12.6448, 33.7826) centre (0, 25.7143) ccw
  spline S15 degree 5 poles (12.6448, 33.7826) (12.6347, 33.7833) (12.6147, 33.7846) (12.5847, 33.7865) (12.5448, 33.7888) (12.4949, 33.7914) (12.4452, 33.7937) (12.3955, 33.7957) (12.3459, 33.7975) (12.2963, 33.7989) (12.2469, 33.8) (12.1975, 33.8009) (12.1483, 33.8014) (12.0991, 33.8017) (12.05, 33.8016) (12.0011, 33.8013) (11.9522, 33.8007) (11.9034, 33.7997) (11.8547, 33.7985) (11.8062, 33.7969) (11.7577, 33.7951) (11.7093, 33.7929) (11.6611, 33.7905) (11.613, 33.7877) (11.565, 33.7846) (11.5171, 33.7813) (11.4693, 33.7776) (11.4217, 33.7735) (11.3741, 33.7692) (11.3267, 33.7646) (11.2795, 33.7596) (11.2324, 33.7543) (11.1854, 33.7487) (11.1385, 33.7428) (11.0918, 33.7366) (11.0453, 33.73) (10.9989, 33.7231) (10.9526, 33.7158) (10.9065, 33.7083) (10.8605, 33.7004) (10.8148, 33.6921) (10.7691, 33.6835) (10.7237, 33.6746) (10.6784, 33.6653) (10.6334, 33.6556) (10.5884, 33.6456) (10.5437, 33.6353) (10.4992, 33.6246) (10.4548, 33.6135) (10.4107, 33.6021) (10.3667, 33.5903) (10.323, 33.5781) (10.2795, 33.5654) (10.2363, 33.5524) (10.1933, 33.5389) (10.1505, 33.5251) (10.108, 33.5108) (10.0656, 33.4962) (10.0235, 33.4813) (9.9817, 33.4659) (9.9402, 33.45) (9.899, 33.4335) (9.8583, 33.4163) (9.818, 33.3985) (9.778, 33.3802) (9.7383, 33.3614) (9.6989, 33.3424) (9.6596, 33.323) (9.6207, 33.3032) (9.5823, 33.2827) (9.5448, 33.2609) (9.5158, 33.242) (9.4947, 33.2269) (9.481, 33.2164) (9.4742, 33.211) knots -1 -1 -1 -1 -1 -1 -0.98571429 -0.97142857 -0.95714286 -0.94285714 -0.92857143 -0.91428571 -0.9 -0.88571429 -0.87142857 -0.85714286 -0.84285714 -0.82857143 -0.81428571 -0.8 -0.78571429 -0.77142857 -0.75714286 -0.74285714 -0.72857143 -0.71428571 -0.7 -0.68571429 -0.67142857 -0.65714286 -0.64285714 -0.62857143 -0.61428571 -0.6 -0.58571429 -0.57142857 -0.55714286 -0.54285714 -0.52857143 -0.51428571 -0.5 -0.48571429 -0.47142857 -0.45714286 -0.44285714 -0.42857143 -0.41428571 -0.4 -0.38571429 -0.37142857 -0.35714286 -0.34285714 -0.32857143 -0.31428571 -0.3 -0.28571429 -0.27142857 -0.25714286 -0.24285714 -0.22857143 -0.21428571 -0.2 -0.18571429 -0.17142857 -0.15714286 -0.14285714 -0.12857143 -0.11428571 -0.1 -0.08571429 -0.07142857 -0.05714286 -0.04285714 -0.02857143 -0.01428571 0 0 0 0 0 0
  line L15 (9.4742, 33.211) -> (8.7021, 32.601)
  arc A31 (7.4859, 32.6935) -> (8.7021, 32.601) centre (8.1441, 33.3073) ccw
  arc A32 (7.4859, 32.6935) -> (6.9792, 33.2001) centre (0, 25.7143) ccw
  arc A33 (6.8868, 34.4163) -> (6.9792, 33.2001) centre (7.593, 33.8584) ccw
  line L16 (6.8868, 34.4163) -> (7.4967, 35.1885)
  spline S16 degree 5 poles (7.4967, 35.1885) (7.5021, 35.1953) (7.5126, 35.209) (7.5277, 35.2301) (7.5466, 35.2591) (7.5684, 35.2966) (7.589, 35.335) (7.6087, 35.3739) (7.6281, 35.4132) (7.6472, 35.4526) (7.6659, 35.4923) (7.6842, 35.5323) (7.702, 35.5726) (7.7192, 35.6133) (7.7357, 35.6545) (7.7516, 35.696) (7.767, 35.7378) (7.782, 35.7799) (7.7966, 35.8223) (7.8108, 35.8648) (7.8246, 35.9076) (7.8381, 35.9506) (7.8511, 35.9938) (7.8638, 36.0373) (7.876, 36.081) (7.8878, 36.125) (7.8992, 36.1691) (7.9103, 36.2135) (7.921, 36.258) (7.9314, 36.3027) (7.9414, 36.3476) (7.951, 36.3927) (7.9603, 36.438) (7.9692, 36.4834) (7.9778, 36.529) (7.9861, 36.5748) (7.994, 36.6208) (8.0016, 36.6669) (8.0088, 36.7131) (8.0157, 36.7596) (8.0223, 36.8061) (8.0285, 36.8528) (8.0345, 36.8997) (8.0401, 36.9466) (8.0453, 36.9938) (8.0503, 37.041) (8.0549, 37.0884) (8.0593, 37.1359) (8.0633, 37.1836) (8.067, 37.2314) (8.0704, 37.2793) (8.0734, 37.3273) (8.0762, 37.3754) (8.0787, 37.4236) (8.0808, 37.472) (8.0827, 37.5204) (8.0842, 37.569) (8.0854, 37.6177) (8.0864, 37.6665) (8.087, 37.7153) (8.0874, 37.7643) (8.0874, 37.8134) (8.0871, 37.8626) (8.0866, 37.9118) (8.0857, 37.9612) (8.0846, 38.0106) (8.0832, 38.0601) (8.0814, 38.1098) (8.0794, 38.1594) (8.0771, 38.2092) (8.0745, 38.2591) (8.0722, 38.299) (8.0703, 38.329) (8.069, 38.349) (8.0683, 38.359) knots 0 0 0 0 0 0 0.01428571 0.02857143 0.04285714 0.05714286 0.07142857 0.08571429 0.1 0.11428571 0.12857143 0.14285714 0.15714286 0.17142857 0.18571429 0.2 0.21428571 0.22857143 0.24285714 0.25714286 0.27142857 0.28571429 0.3 0.31428571 0.32857143 0.34285714 0.35714286 0.37142857 0.38571429 0.4 0.41428571 0.42857143 0.44285714 0.45714286 0.47142857 0.48571429 0.5 0.51428571 0.52857143 0.54285714 0.55714286 0.57142857 0.58571429 0.6 0.61428571 0.62857143 0.64285714 0.65714286 0.67142857 0.68571429 0.7 0.71428571 0.72857143 0.74285714 0.75714286 0.77142857 0.78571429 0.8 0.81428571 0.82857143 0.84285714 0.85714286 0.87142857 0.88571429 0.9 0.91428571 0.92857143 0.94285714 0.95714286 0.97142857 0.98571429 1 1 1 1 1 1
  arc A34 (8.0683, 38.359) -> (6.9165, 39.0241) centre (0, 25.7143) ccw
  spline S17 degree 5 poles (6.9165, 39.0241) (6.9075, 39.0196) (6.8895, 39.0107) (6.8626, 38.9974) (6.8269, 38.9794) (6.7824, 38.9567) (6.7381, 38.9338) (6.6941, 38.9107) (6.6502, 38.8874) (6.6066, 38.8639) (6.5632, 38.8402) (6.5201, 38.8163) (6.4771, 38.7921) (6.4344, 38.7677) (6.392, 38.7432) (6.3497, 38.7184) (6.3077, 38.6934) (6.2659, 38.6682) (6.2244, 38.6428) (6.1831, 38.6172) (6.1421, 38.5913) (6.1013, 38.5653) (6.0607, 38.539) (6.0204, 38.5126) (5.9804, 38.4859) (5.9406, 38.459) (5.9011, 38.4319) (5.8618, 38.4046) (5.8228, 38.3771) (5.7841, 38.3494) (5.7457, 38.3215) (5.7075, 38.2934) (5.6696, 38.265) (5.632, 38.2365) (5.5947, 38.2077) (5.5576, 38.1787) (5.5209, 38.1495) (5.4845, 38.1201) (5.4483, 38.0905) (5.4125, 38.0607) (5.3769, 38.0307) (5.3417, 38.0004) (5.3068, 37.97) (5.2723, 37.9393) (5.2381, 37.9084) (5.2042, 37.8773) (5.1706, 37.8459) (5.1374, 37.8144) (5.1045, 37.7826) (5.072, 37.7507) (5.0399, 37.7185) (5.0081, 37.686) (4.9768, 37.6533) (4.9459, 37.6204) (4.9153, 37.5873) (4.8852, 37.5539) (4.8555, 37.5203) (4.8261, 37.4865) (4.7971, 37.4525) (4.7686, 37.4182) (4.7406, 37.3837) (4.7132, 37.3488) (4.6865, 37.3136) (4.6605, 37.278) (4.635, 37.2422) (4.6101, 37.2061) (4.5854, 37.1698) (4.5611, 37.1335) (4.5373, 37.0969) (4.5143, 37.0599) (4.4928, 37.0223) (4.4771, 36.9914) (4.4664, 36.9678) (4.4597, 36.9518) (4.4565, 36.9437) knots -1 -1 -1 -1 -1 -1 -0.98571429 -0.97142857 -0.95714286 -0.94285714 -0.92857143 -0.91428571 -0.9 -0.88571429 -0.87142857 -0.85714286 -0.84285714 -0.82857143 -0.81428571 -0.8 -0.78571429 -0.77142857 -0.75714286 -0.74285714 -0.72857143 -0.71428571 -0.7 -0.68571429 -0.67142857 -0.65714286 -0.64285714 -0.62857143 -0.61428571 -0.6 -0.58571429 -0.57142857 -0.55714286 -0.54285714 -0.52857143 -0.51428571 -0.5 -0.48571429 -0.47142857 -0.45714286 -0.44285714 -0.42857143 -0.41428571 -0.4 -0.38571429 -0.37142857 -0.35714286 -0.34285714 -0.32857143 -0.31428571 -0.3 -0.28571429 -0.27142857 -0.25714286 -0.24285714 -0.22857143 -0.21428571 -0.2 -0.18571429 -0.17142857 -0.15714286 -0.14285714 -0.12857143 -0.11428571 -0.1 -0.08571429 -0.07142857 -0.05714286 -0.04285714 -0.02857143 -0.01428571 0 0 0 0 0 0
  line L17 (4.4565, 36.9437) -> (4.0928, 36.0294)